Autodesk Fusion 360 part; units mm, degrees
(part 3 of 3)
  spline S558 degree 2 poles (45.7873, -27.9841) (45.3257, -27.7143) (45.065, -27.2048) knots 0 0 0 1 1 1
  spline S559 degree 2 poles (45.065, -27.2048) (44.8042, -26.6952) (44.8042, -26.0358) knots 0 0 0 1 1 1
  spline S560 degree 2 poles (44.8042, -26.0358) (44.8042, -24.5312) (45.7873, -23.9977) knots 0 0 0 1 1 1
  line L371 (45.7873, -23.9977) -> (45.7873, -23.8358)
  spline S561 degree 2 poles (45.7873, -23.8358) (45.3198, -23.5661) (45.062, -23.0415) knots 0 0 0 1 1 1
  spline S562 degree 2 poles (45.062, -23.0415) (44.8042, -22.517) (44.8042, -21.8576) knots 0 0 0 1 1 1
  spline S563 degree 2 poles (44.8042, -21.8576) (44.8042, -20.7187) (45.3887, -20.1342) knots 0 0 0 1 1 1
  spline S564 degree 2 poles (45.3887, -20.1342) (45.9732, -19.5497) (47.262, -19.5497) knots 0 0 0 1 1 1
  line L372 (47.262, -19.5497) -> (51.632, -19.5497)
  line L373 (51.632, -19.5497) -> (51.632, -21.3841)
  line L374 (51.632, -21.3841) -> (47.7176, -21.3841)
  spline S565 degree 2 poles (47.7176, -21.3841) (46.9922, -21.3841) (46.6296, -21.6268) knots 0 0 0 1 1 1
  spline S566 degree 2 poles (46.6296, -21.6268) (46.2669, -21.8696) (46.2669, -22.3911) knots 0 0 0 1 1 1
  spline S567 degree 2 poles (46.2669, -22.3911) (46.2669, -23.0625) (46.7465, -23.3952) knots 0 0 0 1 1 1
  spline S568 degree 2 poles (46.7465, -23.3952) (47.226, -23.7279) (48.2691, -23.7279) knots 0 0 0 1 1 1
  line L375 (48.2691, -23.7279) -> (51.632, -23.7279)
  dimension "d221" = 0.6
  dimension "d223" = 0.6
  constraint horizontal L4
  constraint vertical L5
  constraint horizontal L6
  constraint vertical L7
  constraint horizontal L311
  constraint vertical L312
  constraint horizontal L313
  constraint vertical L314
  measures "d221" distance of L5 L7
  measures "d223" distance of L312 L314
extrude "Extrude39" cut sketch "Sketch71" against normal blind 0.5 contours L4 L5 L6 L7 | L8 L9 L10 L11 L12 L13 S0 S1 S2 L14 | L15 L16 S3 S4 S5 S6 S7 S8 S9 L17 S10 S11 S12 S13 S14 S15 L18 L19 L20 | L21 L22 L23 L24 L25 L26 L27 L28 | S23 S24 L33 L34 L35 L36 L37 S25 S26 | S27 S28 S29 L38 S30 S31 S32 S33 S34 S35 S36 S37 S38 S39 S40 S41 S42 S43 L39 S44 S45 S46 S47 S48 S49 S50 S51 S52 | L40 L41 L42 L43 | L44 L45 L46 S53 S54 S55 S56 S57 S58 S59 L47 S60 S61 S62 S63 S64 S65 S66 S67 S68 L48 L49 L50 L51 | L52 L53 L54 L55 L56 L57 L58 L59 L60 L61 L62 L63 | S69 S70 L64 L65 L66 S71 S72 | L70 L71 S75 L72 L73 L74 L75 L76 L77 L78 L79 L80 L81 L82 S76 S77 L83 L84 L85 | L86 L87 L88 L89 | L90 S78 S79 S80 S81 S82 L91 L92 L93 S83 S84 S85 S86 L94 L95 | S87 S88 S89 L96 S90 S91 S92 S93 S94 S95 S96 S97 S98 S99 S100 S101 S102 S103 L97 S104 S105 S106 S107 S108 S109 S110 S111 S112 | L98 S113 S114 S115 S116 L99 S117 S118 S119 S120 L100 L101 | S128 S129 L108 L109 L110 S130 S131 | L114 L115 L116 L117 L118 L119 L120 L121 S134 S135 S136 L122 S137 S138 S139 L123 L124 L125 | S140 L126 S141 S142 S143 L127 L128 L129 L130 L131 L132 L133 L134 L135 L136 L137 S144 S145 | L141 L142 L143 L144 S150 S151 S152 S153 S154 L145 L146 L147 | S155 S156 S157 S158 L148 S159 S160 S161 S162 S163 S164 S165 S166 S167 S168 S169 S170 L149 S171 S172 S173 S174 S175 S176 S177 S178 | S179 L150 S180 S181 S182 L151 L152 L153 L154 L155 L156 L157 L158 L159 L160 L161 S183 S184 | S189 S190 L165 L166 L167 L168 L169 S191 S192 | S201 S202 S203 S204 S205 S206 S207 S208 S209 S210 | L170 L171 L172 L173 L174 L175 L176 L177 S211 L178 S212 L179 L180 L181 L182 S213 S214 S215 S216 L183 S217 S218 L184 L185 L186 L187 | S223 S224 S225 S226 S227 S228 L189 L190 S229 S230 S231 S232 L191 S233 S234 | S235 L192 S236 S237 S238 L193 L194 L195 L196 L197 L198 S239 S240 | L199 S241 S242 S243 S244 S245 L200 L201 L202 S246 S247 S248 S249 L203 L204 | S250 S251 S252 L205 S253 S254 S255 S256 S257 S258 S259 S260 S261 S262 S263 S264 S265 S266 L206 S267 S268 S269 S270 S271 S272 S273 S274 S275 | L207 S276 S277 S278 S279 L208 S280 S281 S282 S283 L209 L210 | S291 S292 L217 L218 L219 S293 S294 | S297 S298 S299 S300 L223 S301 S302 S303 S304 S305 S306 S307 L224 S308 S309 | L225 L226 L227 L228 L229 L230 L231 L232 | L233 L234 L235 L236 L237 L238 L239 L240 | L241 L242 L243 L244 L245 L246 | L250 L251 L252 L253 S314 S315 S316 S317 S318 L254 L255 L256 | S319 S320 S321 L257 S322 S323 S324 S325 S326 S327 S328 S329 S330 S331 S332 S333 S334 S335 L258 S336 S337 S338 S339 S340 S341 S342 S343 S344 | L259 L260 L261 S345 S346 S347 S348 S349 S350 S351 L262 S352 S353 S354 S355 S356 S357 S358 S359 S360 L263 L264 L265 L266 | S361 S362 L267 S363 S364 S365 S366 S367 L268 S368 S369 S370 S371 S372 S373 L269 L270 L271 S374 S375 S376 S377 S378 L272 S379 S380 S381 | L273 L274 L275 S382 S383 S384 S385 S386 S387 S388 L276 S389 S390 S391 S392 S393 S394 S395 S396 S397 L277 L278 L279 L280 | S398 S399 S400 L281 S401 S402 S403 S404 S405 S406 S407 S408 S409 S410 S411 S412 S413 S414 L282 S415 S416 S417 S418 S419 S420 S421 S422 S423 | S428 S429 S430 S431 S432 S433 L284 L285 S434 S435 S436 S437 L286 S438 S439 | S440 L287 S441 S442 S443 L288 L289 L290 L291 L292 L293 S444 S445 | S446 S447 S448 S449 S450 | L294 L295 L296 L297 | L298 L299 S451 S452 S453 S454 S455 S456 L300 L301 S457 S458 L302 S459 S460 S461 L303 L304 | L307 L308 L309 L310 | L311 L312 L313 L314 | L315 L316 L317 L318 L319 L320 S467 S468 S469 L321 | S474 S475 S476 S477 S478 S479 L323 L324 S480 S481 S482 S483 L325 S484 S485 | S486 L326 S487 S488 S489 L327 L328 L329 L330 L331 L332 S490 S491 | S492 S493 S494 S495 L333 S496 S497 S498 S499 S500 S501 S502 S503 S504 S505 S506 S507 L334 S508 S509 S510 S511 S512 S513 S514 S515 | L335 L336 S516 S517 S518 S519 S520 S521 L337 L338 S522 S523 L339 S524 S525 S526 L340 L341 | L344 L345 L346 L347 L348 L349 L350 L351 | S536 S537 S538 S539 S540 S541 L353 L354 S542 S543 S544 S545 L355 S546 S547 | S548 L356 S549 S550 S551 L357 L358 L359 L360 L361 L362 S552 S553 | L363 L364 S554 S555 S556 S557 L365 L366 L367 L368 L369 L370 S558 S559 S560 L371 S561 S562 S563 S564 L372 L373 L374 S565 S566 S567 S568 L375 bodies 1
extrude "Extrude40" add 56 faces at (5.9646, 89.4799, 0.5) (5.279, 87.4864, 0.5) (5.9406, 82.3191, 0.5) (5.9756, 51.2792, 0.5) (7.6459, 57.3957, 0.5) (6.7255, 60.0705, 0.5) (3.822, 62.8007, 0.5) (6.6694, 43.1987, 0.5) (5.8333, 41.0035, 0.5) (5.3715, 31.5881, 0.5) (6.0687, 26.4654, 0.5) (6.2969, 9.3982, 0.5) (7.6282, 13.155, 0.5) (5.8086, 14.9317, 0.5) (36.5175, 5.7147, 0.5) (39.434, 5.6797, 0.5) (44.625, 6.4423, 0.5) (50.6526, 5.6797, 0.5) (53.1913, 4.9105, 0.5) (58.5592, 5.8007, 0.5) (47.5277, 79.1436, 0.5) (48.331, 72.2578, 0.5) (48.2611, 68.1495, 0.5) (48.5079, 61.012, 0.5) (49.3572, 52.1576, 0.5) (49.2262, 47.3804, 0.5) (48.331, 38.8022, 0.5) (48.2611, 34.694, 0.5) (48.347, 29.119, 0.5) (79.4737, 90.1521, 0.5) (81.7805, 86.7438, 0.5) (81.7424, 84.503, 0.5) (81.144, 81.1297, 0.5) (78.981, 81.562, 0.5) (82.3402, 77.0651, 0.5) (80.1892, 75.0414, 0.5) (88.6235, 92.39, 0.5) (86.9957, 86.0578, 0.5) (90.8197, 83.4189, 0.5) (88.6221, 79.3454, 0.5) (90.8197, 75.7742, 0.5) (84.7897, 56.1254, 0.5) (89.1555, 51.6514, 0.5) (89.7157, 54.6988, 0.5) (89.7157, 58.5768, 0.5) (87.1335, 5.4335, 0.5) (89.3385, 12.991, 0.5) (84.7763, 21.1346, 0.5) (88.9076, 20.2965, 0.5) (87.088, 22.0732, 0.5) (88.4193, 25.83, 0.5) (81.657, 25.1727, 0.5) (81.2497, 29.0887, 0.5) (81.7892, 20.7934, 0.5) (81.8862, 13.3743, 0.5) (81.8481, 11.1334, 0.5) along direction (0, 0, -1) blind 0.5 separate body on bodies 1 makes body 3 at (81.8862, 13.3743, 0.5) makes body 4 at (81.2497, 29.0887, 0.5) makes body 5 at (88.4193, 25.83, 0.5) makes body 6 at (88.9076, 20.2965, 0.5) makes body 7 at (89.3385, 12.991, 0.5) makes body 8 at (89.7157, 58.5768, 0.5) makes body 9 at (89.1555, 51.6514, 0.5) makes body 10 at (90.8197, 75.7742, 0.5) makes body 11 at (90.8197, 83.4189, 0.5) makes body 12 at (88.6235, 92.39, 0.5) makes body 13 at (82.3402, 77.0651, 0.5) makes body 14 at (81.144, 81.1297, 0.5) makes body 15 at (81.7805, 86.7438, 0.5) makes body 16 at (48.347, 29.119, 0.5) makes body 17 at (48.331, 38.8022, 0.5) makes body 18 at (49.3572, 52.1576, 0.5) makes body 19 at (48.2611, 68.1495, 0.5) makes body 20 at (47.5277, 79.1436, 0.5) makes body 21 at (53.1913, 4.9105, 0.5) makes body 22 at (44.625, 6.4423, 0.5) makes body 23 at (36.5175, 5.7147, 0.5) makes body 24 at (7.6282, 13.155, 0.5) makes body 25 at (6.0687, 26.4654, 0.5) makes body 26 at (5.8333, 41.0035, 0.5) makes body 27 at (3.822, 62.8007, 0.5) makes body 28 at (7.6459, 57.3957, 0.5) makes body 29 at (5.9406, 82.3191, 0.5) makes body 30 at (5.9646, 89.4799, 0.5) makes body 31 at (5.279, 87.4864, 0.5) makes body 32 at (5.9756, 51.2792, 0.5) makes body 33 at (6.7255, 60.0705, 0.5) makes body 34 at (6.6694, 43.1987, 0.5) makes body 35 at (5.3715, 31.5881, 0.5) makes body 36 at (6.2969, 9.3982, 0.5) makes body 37 at (5.8086, 14.9317, 0.5) makes body 38 at (39.434, 5.6797, 0.5) makes body 39 at (50.6526, 5.6797, 0.5) makes body 40 at (58.5592, 5.8007, 0.5) makes body 41 at (48.331, 72.2578, 0.5) makes body 42 at (48.5079, 61.012, 0.5) makes body 43 at (49.2262, 47.3804, 0.5) makes body 44 at (48.2611, 34.694, 0.5) makes body 45 at (79.4737, 90.1521, 0.5) makes body 46 at (81.7424, 84.503, 0.5) makes body 47 at (78.981, 81.562, 0.5) makes body 48 at (80.1892, 75.0414, 0.5) makes body 49 at (86.9957, 86.0578, 0.5) makes body 50 at (88.6221, 79.3454, 0.5) makes body 51 at (84.7897, 56.1254, 0.5) makes body 52 at (89.7157, 54.6988, 0.5) makes body 53 at (87.1335, 5.4335, 0.5) makes body 54 at (84.7763, 21.1346, 0.5) makes body 55 at (87.088, 22.0732, 0.5) makes body 56 at (81.657, 25.1727, 0.5) makes body 57 at (81.7892, 20.7934, 0.5) makes body 58 at (81.8481, 11.1334, 0.5)
